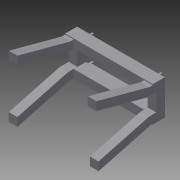
# Autodesk Inventor part: jembutrangka
Saved by Autodesk Inventor 2013 (Build 170138000, 138)
## iProperties
Created: 2016-04-02
Part Number: jembutrangka
Material: Generic
Document SubType Name: Modeling
Designer: yuyudhn
Density: 1 g/cm^3
Author: yuyudhn
Autodesk Inventor part; units mm, degrees
ref_plane "YZ Plane" through (0, 0, 0) normal (1, 0, 0) x (0, 1, 0)
ref_plane "XZ Plane" through (0, 0, 0) normal (0, 1, 0) x (-1, 0, 0)
ref_plane "XY Plane" through (0, 0, 0) normal (0, 0, 1) x (1, 0, 0)
sketch "Sketch1" plane through (0, 0, 0) normal (0, 1, 0) x (-1, 0, 0)
  line L0 (0, 0) -> (50000, 0)
  line L1 (50000, 0) -> (50000, -20000)
  line L2 (50000, -20000) -> (0, -20000)
  line L3 (0, -20000) -> (0, 0)
  dimension "d0" = 50000
  dimension "d1" = 20000
  constraints: 8 end point, 2 parallel, 1 horizontal, 1 perpendicular
  measures "d0" distance of L1.end L2.end
  measures "d1" distance of L0.end L1.end
extrude "Extrusion1" add sketch "Sketch1" along normal blind 7000
sketch "Sketch2" plane through (0, 7000, 0) normal (0, 1, 0) x (1, 0, 0)
  line L0 (-50000, 0) -> (0, 0) projected
  line L1 (0, 0) -> (0, 20000) projected
  line L2 (0, 20000) -> (-50000, 20000) projected
  line L3 (-50000, 20000) -> (-50000, 0) projected
  line L4 (-45094.1983, 15094.1983) -> (-4905.8017, 15094.1983)
  line L5 (-4905.8017, 15094.1983) -> (-4905.8017, 4905.8017)
  line L6 (-4905.8017, 4905.8017) -> (-45094.1983, 4905.8017)
  line L7 (-45094.1983, 4905.8017) -> (-45094.1983, 15094.1983)
  constraints: 8 end point, 3 other
extrude "Extrusion2" cut sketch "Sketch2" against normal blind 7000 contours L4 L5 L6 L7
sketch "Sketch3" plane through (-50000, 0, -20000) normal (-1, 0, 0) x (0, 0, 1)
  line L0 (20000, 0) -> (0, 0) projected
  line L1 (10000, 0) -> (15000, 0)
  line L2 (15000, 0) -> (15000, 2000)
  line L3 (15000, 2000) -> (10000, 2000)
  line L4 (10000, 0) -> (5000, 0)
  line L5 (5000, 0) -> (5000, 2000)
  line L6 (5000, 2000) -> (10000, 2000)
  dimension "d6" = 5000
  dimension "d7" = 2000
  constraints: 12 end point, 1 horizontal, 1 midpoint, 1 parallel, 1 perpendicular
  measures "d6" distance of L3.end L2.end
  measures "d7" distance of L2.end L1.end
extrude "Extrusion3" cut sketch "Sketch3" against normal blind 997000
sketch "Sketch6" plane through (0, 0, 0) normal (0, -1, 0) x (1, 0, 0)
  line L0 (-50000, -15000) -> (-45094.1983, -15000)
  line L1 (-45094.1983, -15000) -> (-45094.1983, -19500)
  line L2 (-45094.1983, -19500) -> (-50000, -19500)
  line L3 (-50000, -19500) -> (-50000, -15000)
  line L4 (0, -15000) -> (-4905.8017, -15000)
  line L5 (-4905.8017, -15000) -> (-4905.8017, -19500)
  line L6 (-4905.8017, -19500) -> (0, -19500)
  line L7 (0, -19500) -> (0, -15000)
  point P0 (0, 0)
  dimension "d14" = 4500
  dimension "d15" = 4500
  constraints: 16 end point, 4 parallel, 2 horizontal, 2 perpendicular
  measures "d14" distance of L0.end L1.end
  measures "d15" distance of L5.end L4.end
extrude "Extrusion6" add sketch "Sketch6" along normal blind 2000
sketch "Sketch7" plane through (0, 0, 0) normal (0, -1, 0) x (1, 0, 0)
  line L0 (-50000, -5000) -> (-45094.1983, -5000)
  line L1 (-45094.1983, -5000) -> (-45094.1983, -500)
  line L2 (-45094.1983, -500) -> (-50000, -500)
  line L3 (-50000, -500) -> (-50000, -5000)
  line L4 (0, -5000) -> (-4905.8017, -5000)
  line L5 (-4905.8017, -5000) -> (-4905.8017, -500)
  line L6 (-4905.8017, -500) -> (0, -500)
  line L7 (0, -500) -> (0, -5000)
  dimension "d18" = 4500
  dimension "d19" = 4500
  constraints: 16 end point, 4 parallel, 2 horizontal, 2 perpendicular
  measures "d18" distance of L1.end L0.end
  measures "d19" distance of L4.end L5.end
extrude "Extrusion7" add sketch "Sketch7" along normal blind 2000
draft "FaceDraft1" angle 15 pull direction (0, 0, 1) fixed plane through (-1635.2672, -666.6667, -500) normal (0, 0, 1) faces at (-1635.2672, -2000, -3500)
draft "FaceDraft2" angle 15 pull direction (0, 0, 1) fixed plane through (-48364.7328, -666.6667, -500) normal (0, 0, 1) faces at (-48364.7328, -2000, -2000)
draft "FaceDraft3" angle 15 pull direction (0, 0, -1) fixed plane through (-46729.4655, -666.6667, -19500) normal (0, 0, -1) faces at (-48364.7328, -2000, -16500)
draft "FaceDraft4" angle 15 pull direction (0, 0, -1) faces at (-3270.5345, -2000, -16500) fixed edges at (-2452.9009, -2000, -15000)
sketch "Sketch8" plane through (-4905.8017, -2000, -15000) normal (0, -0.9659258, -0.258819) x (1, 0, 0)
  line L0 (4905.8017, 0) -> (0, 0) projected
  line L1 (0, 0) -> (0, -4658.7428) projected
  line L2 (0, -4658.7428) -> (4905.8017, -4658.7428) projected
  line L3 (4905.8017, -4658.7428) -> (4905.8017, 0) projected
  point P0 (4905.8017, 13971.2493)
extrude "Extrusion8" add sketch "Sketch8" along normal blind 30000
sketch "Sketch9" plane through (-50000, -2000, -19500) normal (0, -0.9659258, -0.258819) x (1, 0, 0)
  line L0 (0, 4658.7428) -> (0, 0) projected
  line L1 (0, 0) -> (4905.8017, 0) projected
  line L2 (4905.8017, 0) -> (4905.8017, 4658.7428) projected
  line L3 (4905.8017, 4658.7428) -> (0, 4658.7428) projected
  point P0 (50000, 18317.9155)
extrude "Extrusion9" add sketch "Sketch9" along normal blind 30000
sketch "Sketch10" plane through (-50000, -3205.7714, -5000) normal (0, -0.9659258, 0.258819) x (1, 0, 0)
  line L0 (0, 0) -> (4905.8017, 0) projected
  line L1 (4905.8017, 0) -> (4905.8017, 4658.7428) projected
  line L2 (4905.8017, 4658.7428) -> (0, 4658.7428) projected
  line L3 (0, 4658.7428) -> (0, 0) projected
  point P0 (50000, 5659.3438)
extrude "Extrusion10" add sketch "Sketch10" along normal blind 30000
sketch "Sketch11" plane through (-4905.8017, -2000, -500) normal (0, -0.9659258, 0.258819) x (1, 0, 0)
  line L0 (4905.8017, -4658.7428) -> (4905.8017, 0) projected
  line L1 (4905.8017, 0) -> (0, 0) projected
  line L2 (0, 0) -> (0, -4658.7428) projected
  line L3 (0, -4658.7428) -> (4905.8017, -4658.7428) projected
  point P0 (4905.8017, 1000.601)
extrude "Extrusion11" add sketch "Sketch11" along normal blind 30000
draft "FaceDraft5" angle 15 pull direction (0, -0.258819, 0.9659258) fixed plane through (-3270.5345, -11659.2583, -17588.1905) normal (0, -0.258819, 0.9659258) faces at (-3270.5345, -30575.851, -24264.5714)
draft "FaceDraft6" angle 15 pull direction (0, -0.258819, -0.9659258) fixed plane through (-3270.5345, -12865.0296, -2411.8095) normal (0, -0.258819, -0.9659258) faces at (-3270.5345, -31781.6224, 4264.5714)
draft "FaceDraft7" angle 15 pull direction (0, -0.258819, 0.9659258) fixed plane through (-48364.7328, -22524.2879, -20176.3809) normal (0, -0.258819, 0.9659258) faces at (-48364.7328, -31379.6986, -25764.5714)
draft "FaceDraft8" angle 15 pull direction (0, -0.258819, -0.9659258) fixed plane through (-46729.4655, -12865.0296, -2411.8095) normal (0, -0.258819, -0.9659258) faces at (-48364.7328, -31379.6986, 5764.5714)
fillet "Fillet1" radius 300 2 edges at (-25000, 7000, -20000) (-25000, 7000, 0)
sketch "Sketch12" plane through (0, 7000, 0) normal (0, 1, 0) x (1, 0, 0)
  line L0 (-45094.1983, 16294.1983) -> (-4905.8017, 16294.1983)
  line L1 (-4905.8017, 16294.1983) -> (-4905.8017, 17794.1983)
  line L2 (-4905.8017, 17794.1983) -> (-45094.1983, 17794.1983)
  line L3 (-45094.1983, 17794.1983) -> (-45094.1983, 16294.1983)
  line L4 (-45094.1983, 3705.8017) -> (-4905.8017, 3705.8017)
  line L5 (-4905.8017, 3705.8017) -> (-4905.8017, 2205.8017)
  line L6 (-4905.8017, 2205.8017) -> (-45094.1983, 2205.8017)
  line L7 (-45094.1983, 2205.8017) -> (-45094.1983, 3705.8017)
  point P0 (-45094.1983, 4905.8017)
  point P1 (-45094.1983, 15094.1983)
  point P2 (0, 0)
  dimension "d39" = 1200
  dimension "d40" = 1500
  dimension "d41" = 1200
  dimension "d42" = 1500
  constraints: 16 end point, 4 parallel, 2 horizontal, 2 perpendicular
  measures "d39" distance of point (-45094.198, 15094.198) L0.start
  measures "d40" distance of L1.end L0.end
  measures "d41" distance of point (-45094.198, 4905.802) L4.start
  measures "d42" distance of L4.end L5.end
extrude "Extrusion12" add sketch "Sketch12" along normal blind 2000
sketch "Sketch13" plane through (0, 9000, 0) normal (0, 1, 0) x (1, 0, 0)
  line L0 (-45094.1983, 2205.8017) -> (-4905.8017, 2205.8017) projected
  line L1 (-45094.1983, 3705.8017) -> (-44094.1983, 3705.8017)
  line L2 (-44094.1983, 3705.8017) -> (-44094.1983, 2205.8017)
  line L3 (-44094.1983, 2205.8017) -> (-45094.1983, 2205.8017)
  line L4 (-45094.1983, 2205.8017) -> (-45094.1983, 3705.8017)
  line L5 (-4905.8017, 3705.8017) -> (-5905.8017, 3705.8017)
  line L6 (-5905.8017, 3705.8017) -> (-5905.8017, 2205.8017)
  line L7 (-5905.8017, 2205.8017) -> (-4905.8017, 2205.8017)
  line L8 (-4905.8017, 2205.8017) -> (-4905.8017, 3705.8017)
  point P0 (0, 0)
  dimension "d45" = 1000
  dimension "d46" = 1000
  constraints: 16 end point, 4 parallel, 2 horizontal, 2 perpendicular, 2 point on line
  measures "d45" distance of L2.end L3.end
  measures "d46" distance of L7.end L6.end
extrude "Extrusion13" add sketch "Sketch13" along normal blind 1500
sketch "Sketch14" plane through (0, 9000, 0) normal (0, 1, 0) x (1, 0, 0)
  line L0 (-45094.1983, 16294.1983) -> (-4905.8017, 16294.1983) projected
  line L1 (-45094.1983, 17794.1983) -> (-44094.1983, 17794.1983)
  line L2 (-44094.1983, 17794.1983) -> (-44094.1983, 16294.1983)
  line L3 (-44094.1983, 16294.1983) -> (-45094.1983, 16294.1983)
  line L4 (-45094.1983, 16294.1983) -> (-45094.1983, 17794.1983)
  line L5 (-4905.8017, 17794.1983) -> (-5905.8017, 17794.1983)
  line L6 (-5905.8017, 17794.1983) -> (-5905.8017, 16294.1983)
  line L7 (-5905.8017, 16294.1983) -> (-4905.8017, 16294.1983)
  line L8 (-4905.8017, 16294.1983) -> (-4905.8017, 17794.1983)
  point P0 (0, 0)
  dimension "d49" = 1000
  dimension "d50" = 1000
  constraints: 16 end point, 4 parallel, 2 horizontal, 2 perpendicular, 2 point on line
  measures "d49" distance of L2.end L3.end
  measures "d50" distance of L7.end L6.end
extrude "Extrusion14" add sketch "Sketch14" along normal blind 1500
body "Solid1"
